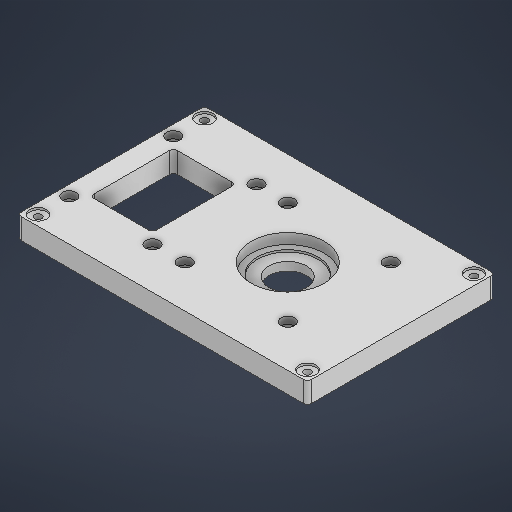
# Autodesk Inventor part: plate for print
Saved by Autodesk Inventor 2025.2 (Build 292293000, 293)
## iProperties
Created: 2025-04-19
Part Number: plate for print
Material: Generic
Document SubType Name: Modeling
Designer: klawy
Density: 1 g/cm^3
Appearance: Default
Author: klawy
Autodesk Inventor part; units mm, degrees
ref_plane "YZ Plane" through (0, 0, 0) normal (1, 0, 0) x (0, 1, 0)
ref_plane "XZ Plane" through (0, 0, 0) normal (0, 1, 0) x (-1, 0, 0)
ref_plane "XY Plane" through (0, 0, 0) normal (0, 0, 1) x (1, 0, 0)
sketch "Sketch1" plane through (0, 0, 0) normal (0, 1, 0) x (-1, 0, 0)
  line L0 (69.75, 45) -> (-69.75, 45)
  line L1 (-69.75, 45) -> (-69.75, -45)
  line L2 (-69.75, -45) -> (69.75, -45)
  line L3 (69.75, -45) -> (69.75, 45)
  line L4 (69.75, 45) -> (-69.75, -45) construction
  line L5 (-69.75, 45) -> (69.75, -45) construction
  circle A0 centre (44.75, 0) radius 8 construction
  circle A1 centre (-15.25, 0) radius 14.5
  line L6 (152.1746, 0) -> (-152.1746, 0) construction
  line L7 (0, 58.0523) -> (0, -58.0523) construction
  line L8 (29.75, 20) -> (59.75, 20)
  line L9 (59.75, 20) -> (59.75, -20)
  line L10 (59.75, -20) -> (29.75, -20)
  line L11 (29.75, -20) -> (29.75, 20)
  line L12 (29.75, 20) -> (59.75, -20) construction
  line L13 (59.75, 20) -> (29.75, -20) construction
  point P0 (0, 0)
  dimension "d0" = 139.5
  dimension "d1" = 16
  dimension "d2" = 29
  dimension "d3" = 25
  dimension "d4" = 90
  dimension "d5" = 54.5
  dimension "d42" = 30
  dimension "d43" = 40
  constraints: 28 end point, 6 midpoint, 4 parallel, 3 horizontal, 2 centre point, 2 perpendicular, 2 point on line, 1 vertical
  measures "d0" distance of L1.end L2.end
  measures "d1" diameter of A0
  measures "d2" diameter of A1
  measures "d3" distance from line of L3 A0.centre
  measures "d4" distance of L0.end L1.end
  measures "d5" distance from line of L1 A1.centre
  measures "d42" distance of L9.end L10.end
  measures "d43" distance of L10.end L8.start
extrude "Extrusion1" add sketch "Sketch1" along normal blind 10
sketch "Sketch2" plane through (0, 0, 0) normal (0, -1, 0) x (1, 0, 0)
  line L0 (64.75, 40) -> (-64.75, 40) construction
  line L1 (-64.75, 40) -> (-64.75, -40) construction
  line L2 (-64.75, -40) -> (64.75, -40) construction
  line L3 (64.75, -40) -> (64.75, 40) construction
  line L4 (64.75, 40) -> (-64.75, -40) construction
  line L5 (-64.75, 40) -> (64.75, -40) construction
  line L6 (69.75, -45) -> (-69.75, -45) construction
  line L7 (-69.75, -45) -> (-69.75, 45) construction
  point P0 (0, 0)
  dimension "d11" = 5
  dimension "d12" = 5
  constraints: 12 end point, 4 coincident, 2 midpoint, 2 parallel, 1 horizontal, 1 perpendicular
  measures "d11" distance between parallel lines of L6 L2
  measures "d12" distance between parallel lines of L7 L1
hole "Hole1" at (64.75, 0, -40) at (-64.75, 0, -40) at (-64.75, 0, 40) at (64.75, 0, 40) direction (0, 1, 0) diameter 3.4 end through all counterbore diameter 6.5 counterbore depth 3.4 clearance for "Socket Head Cap Screw ISO 4762" size "M3" standard "ISO"
sketch "Sketch3" plane through (0, 10, 0) normal (0, 1, 0) x (1, 0, 0)
  circle A0 centre (-64.75, 40) radius 1.7 projected
  circle A1 centre (-64.75, 40) radius 4
  circle A2 centre (64.75, -40) radius 1.7 projected
  circle A3 centre (-64.75, -40) radius 1.7 projected
  circle A4 centre (-64.75, 40) radius 1.7 projected
  circle A5 centre (64.75, 40) radius 1.7 projected
  line L0 (69.75, -45) -> (69.75, 45) projected
  line L1 (69.75, 45) -> (-69.75, 45) projected
  line L2 (-69.75, 45) -> (-69.75, -45) projected
  line L3 (-69.75, -45) -> (69.75, -45) projected
  circle A6 centre (64.75, 40) radius 4
  circle A7 centre (-64.75, -40) radius 4
  circle A8 centre (64.75, -40) radius 4
  point P0 (0, 0)
  dimension "d22" = 129.5
  dimension "d25" = 80
  dimension "d28" = 8
  dimension "d37" = 90
  dimension "d38" = 139.5
  constraints: 4 centre point, 1 coincident, 1 horizontal, 1 vertical, 6 other
  measures "d22" distance of A1.centre A6.centre
  measures "d25" distance of A1.centre A7.centre
  measures "d28" diameter of A1
  measures "d37" distance of L1.end L2.end
  measures "d38" distance of L0.end L1.end
extrude "Extrusion2" cut sketch "Sketch3" against normal blind 1 contours A0 | A1 | A2 | A3 | A5 | A6 | A7 | A8
sketch "Sketch4" plane through (0, 10, 0) normal (0, 1, 0) x (1, 0, 0)
  circle A0 centre (-64.75, 40) radius 4 projected
  line L0 (69.75, -45) -> (69.75, 45) projected
  line L1 (69.75, 45) -> (-69.75, 45) projected
  line L2 (-69.75, 45) -> (-69.75, -45) projected
  line L3 (-69.75, -45) -> (69.75, -45) projected
  circle A1 centre (15.25, 0) radius 14.5 projected
  circle A2 centre (15.25, 0) radius 17.5
  point P0 (0, 0)
  dimension "d31" = 35
  constraints: 1 centre point, 1 coincident
  measures "d31" diameter of A2
extrude "Extrusion3" cut sketch "Sketch4" against normal blind 5 contours A2
sketch "Sketch5" plane through (0, 0, 0) normal (0, -1, 0) x (1, 0, 0)
  circle A0 centre (15.25, 0) radius 14.5 projected
  line L0 (69.75, 45) -> (69.75, -45) projected
  line L1 (-69.75, 45) -> (69.75, 45) projected
  line L2 (-69.75, -45) -> (-69.75, 45) projected
  line L3 (69.75, -45) -> (-69.75, -45) projected
  circle A1 centre (64.75, -40) radius 3.25 projected
  circle A2 centre (-64.75, -40) radius 3.25 projected
  circle A3 centre (-64.75, 40) radius 3.25 projected
  circle A4 centre (64.75, 40) radius 3.25 projected
  circle A5 centre (15.25, 0) radius 9
  point P0 (0, 0)
  dimension "d39" = 18
  constraints: 1 centre point, 1 coincident
  measures "d39" diameter of A5
extrude "Extrusion4" add sketch "Sketch5" against normal blind 4 contours A0
fillet "Fillet1" radius 2 8 edges at (-69.75, 5, 45) (69.75, 5, 45) (69.75, 5, -45) (-69.75, 5, -45) (-59.75, 5, 20) (-59.75, 5, -20) (-29.75, 5, -20) (-29.75, 5, 20)
sketch "Sketch7" plane through (0, 10, 0) normal (0, 1, 0) x (1, 0, 0)
  circle A0 centre (15.25, 0) radius 17.5 projected
  line L0 (15.25, 0) -> (53.4324, -38.1824) construction
  line L1 (-97.65, 0) -> (97.65, 0) projected
  point P0 (0, 0)
  point P1 (39.9987, -24.7487)
  point P2 (39.9987, 24.7487)
  point P3 (-9.4987, 24.7487)
  point P4 (-9.4987, -24.7487)
  dimension "d46" = 35
  dimension "d49" = 360
  dimension "d51" = 45
  constraints: 2 end point, 1 point on line, 5 other
  measures "d46" distance of L0.start point (39.999, -24.749)
  measures "d51" angle of L1 L0
hole "Hole2" at (39.9987, 10, 24.7487) at (39.9987, 10, -24.7487) at (-9.4987, 10, -24.7487) at (-9.4987, 10, 24.7487) direction (0, -1, 0) diameter 3.4 end through all counterbore diameter 6.5 counterbore depth 3.4 clearance for "Socket Head Cap Screw ISO 4762" size "M3" standard "ISO"
sketch "Sketch9" plane through (0, 10, 0) normal (0, 1, 0) x (1, 0, 0)
  line L0 (-57.75, 20) -> (-31.75, 20) construction
  line L1 (-59.75, -18) -> (-59.75, 18) construction
  line L2 (-31.75, -20) -> (-57.75, -20) construction
  line L3 (-29.75, 18) -> (-29.75, -18) construction
  line L4 (-64.75, 25) -> (-24.75, 25) construction
  line L5 (-24.75, 25) -> (-24.75, -25) construction
  line L6 (-24.75, -25) -> (-64.75, -25) construction
  line L7 (-64.75, -25) -> (-64.75, 25) construction
  point P0 (0, 0)
  dimension "d63" = 5
  dimension "d64" = 5
  dimension "d65" = 5
  dimension "d66" = 5
  constraints: 8 end point, 4 coincident, 2 parallel, 1 horizontal, 1 perpendicular
  measures "d63" distance between parallel lines of L4 L0
  measures "d64" distance between parallel lines of L7 L1
  measures "d65" distance between parallel lines of L6 L2
  measures "d66" distance between parallel lines of L3 L5
hole "Hole3" at (-64.75, 10, -25) at (-24.75, 10, -25) at (-24.75, 10, 25) at (-64.75, 10, 25) direction (0, -1, 0) diameter 3.4 end through all counterbore diameter 6.5 counterbore depth 3.4 clearance for "Socket Head Cap Screw ISO 4762" size "M3" standard "ISO"
body "Solid1"
